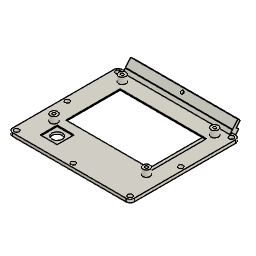
Display Mount Mini - LCD12864 Stock (Autodesk Fusion 360 design; units mm, degrees)
Autodesk Fusion 360 part; units mm, degrees
sketch "Sketch1" plane through (0, 0, 0) normal (0, 0, 1) x (1, 0, 0)
  line L0 (-57.9, 52.128) -> (57.9, 52.128)
  line L1 (57.9, 52.128) -> (57.9, -52.128)
  line L2 (57.9, -52.128) -> (-57.9, -52.128)
  line L3 (-57.9, -52.128) -> (-57.9, 52.128)
  circle A0 centre (-54, 48.228) radius 3.9
  circle A1 centre (-54, 0) radius 2.25
  circle A2 centre (-54, -48.228) radius 3.9
  circle A3 centre (0, -48.228) radius 2.25
  circle A4 centre (54, -48.228) radius 3.9
  circle A5 centre (54, 0) radius 2.25
  circle A6 centre (54, 48.228) radius 3.9
  circle A7 centre (-54, 48.228) radius 2.25
  circle A8 centre (-54, -48.228) radius 2.25
  circle A9 centre (54, -48.228) radius 2.25
  circle A10 centre (54, 48.228) radius 2.25
  point P0 (0, 52.128)
  point P1 (-57.9, 0)
  dimension "d1" = 115.8
  dimension "d2" = 104.256
  dimension "d3" = 7.8
  dimension "d4" = 7.8
  dimension "d5" = 7.8
  dimension "d6" = 7.8
  dimension "d7" = 4.5
  dimension "d8" = 4.5
  dimension "d9" = 4.5
  dimension "d10" = 4.5
  dimension "d11" = 4.5
  dimension "d12" = 4.5
  dimension "d13" = 4.5
  dimension "d14" = 48.128
  dimension "d15" = 96.256
  dimension "d16" = 53.9
  dimension "d17" = 107.8
  constraint horizontal L0
  constraint vertical L1
  constraint horizontal L2
  constraint vertical L3
  constraint midpoint L0 P0
  constraint midpoint L3 P1
  constraint vertical origin P0
  constraint horizontal origin P1
  constraint concentric A0 A7
  constraint concentric A2 A8
  constraint concentric A4 A9
  constraint concentric A6 A10
  constraint tangent L0 A0
  constraint tangent L3 A0
  constraint tangent L1 A4
  constraint tangent L2 A4
  constraint horizontal A0.centre A6.centre
  constraint vertical A5.centre A6.centre
  constraint vertical A5.centre A4.centre
  constraint horizontal A3.centre A2.centre
  constraint horizontal A3.centre A4.centre
  constraint vertical A1.centre A0.centre
  constraint vertical A1.centre A2.centre
  constraint horizontal origin A1.centre
  constraint horizontal origin A5.centre
  constraint vertical origin A3.centre
  measures "d1" distance of L1.end L2.end
  measures "d2" distance of L0.end L1.end
  measures "d3" diameter of A0
  measures "d4" diameter of A2
  measures "d5" diameter of A4
  measures "d6" diameter of A6
  measures "d7" diameter of A1
  measures "d8" diameter of A5
  measures "d9" diameter of A3
  measures "d10" diameter of A7
  measures "d11" diameter of A8
  measures "d12" diameter of A9
  measures "d13" diameter of A10
extrude "Extrude1" add sketch "Sketch1" along normal blind 3 contours L0 L1 L2 L3 A0 A2 A4 A6 | A0 | A6 | A2 | A4
sketch "Sketch2" plane through (0, 0, 0) normal (1, 0, 0) x (0, 1, 0)
  line L0 (-2.25, 3) -> (2.25, 3)
  line L1 (-50.478, 3) -> (-45.978, 3)
  line L2 (-2.25, 3) -> (2.25, 3)
  line L3 (45.978, 3) -> (50.478, 3)
  line L4 (-50.478, 3) -> (-45.978, 3)
  line L5 (45.978, 3) -> (50.478, 3)
  line L6 (-50.478, 3) -> (-45.978, 3)
  line L7 (-48.228, 3) -> (-52.128, 3)
  line L8 (-48.228, 3) -> (48.228, 3)
  line L9 (52.128, 3) -> (48.228, 3)
  line L10 (52.128, 3) -> (48.228, 3)
  line L11 (48.228, 3) -> (-48.228, 3)
  line L12 (-48.228, 3) -> (-52.128, 3)
  line L13 (52.128, 0) -> (52.128, 3)
  line L14 (52.128, 3) -> (52.128, 0)
  line L15 (-2.25, 0) -> (2.25, 0)
  line L16 (-50.478, 0) -> (-45.978, 0)
  line L17 (-2.25, 0) -> (2.25, 0)
  line L18 (45.978, 0) -> (50.478, 0)
  line L19 (-50.478, 0) -> (-45.978, 0)
  line L20 (45.978, 0) -> (50.478, 0)
  line L21 (-50.478, 0) -> (-45.978, 0)
  line L22 (-48.228, 0) -> (-52.128, 0)
  line L23 (-48.228, 0) -> (-52.128, 0)
  line L24 (-48.228, 0) -> (48.228, 0)
  line L25 (52.128, 0) -> (48.228, 0)
  line L26 (52.128, 0) -> (48.228, 0)
  line L27 (48.228, 0) -> (-48.228, 0)
  line L28 (52.128, 3) -> (52.128, 6)
  line L29 (52.128, 6) -> (55.128, 6)
  line L30 (55.128, 6) -> (58.0826, 3.5208)
  line L31 (58.0826, 3.5208) -> (56.1543, 1.2226)
  line L32 (56.1543, 1.2226) -> (62.2826, -3.9197)
  line L33 (62.2826, -3.9197) -> (61.2567, -5.1423)
  line L34 (61.2567, -5.1423) -> (55.1284, 0)
  line L35 (56.1543, 1.2226) -> (55.1284, 0)
  line L36 (55.1284, 0) -> (52.128, 0)
  dimension "d20" = 3
  dimension "d21" = 3
  dimension "d22" = 140
  dimension "d24" = 3.857
  dimension "d26" = 3
  dimension "d27" = 8
  dimension "d28" = 1.596
  constraint coincident L9.start L10.start
  constraint perpendicular L10 L28
  constraint perpendicular L28 L29
  constraint perpendicular L30 L31
  constraint perpendicular L31 L32
  constraint perpendicular L32 L33
  constraint perpendicular L33 L34
  constraint collinear L31 L35
  constraint coincident L13.start L14.end
  measures "d20" distance of L9.start L28.end
  measures "d21" distance of L28.end L29.end
  measures "d22" angle of L29 L30
  measures "d24" distance of L29.end L30.end
  measures "d26" distance of L30.end L31.end
  measures "d27" distance of L31.end L32.end
  measures "d28" distance of L32.end L33.end
extrude "Extrude2" add sketch "Sketch2" along normal mid plane 102 contours L13 L14 L28 L29 L30 L31 L35 L36
sketch "Sketch1 (2)" plane through (0, 25.732, 30.6662) normal (0, 0.642788, 0.766044) x (-1, 0, 0)
  line L0 (51, -38.3738) -> (-51, -38.3738)
  line L1 (-51, -38.3738) -> (-51, -42.2308)
  line L2 (-51, -42.2308) -> (51, -42.2308)
  line L3 (51, -42.2308) -> (51, -38.3738)
  line L4 (51, -39.2308) -> (-51, -39.2308)
  line L5 (-51, -39.2308) -> (-51, -36.2308)
  line L6 (-51, -36.2308) -> (51, -36.2308)
  line L7 (51, -36.2308) -> (51, -39.2308)
  dimension "d67" = 3
  dimension "d68" = 3
  constraint horizontal L4
  constraint vertical L5
  constraint horizontal L6
  constraint vertical L7
  constraint collinear L1 L5
  constraint collinear L3 L7
  measures "d67" distance of L2 L4
  measures "d68" distance of L4 L6
extrude "Extrude4" add sketch "Sketch1 (2)" against normal blind 7 contours L0 L1 L3 L4 L5 L7 | L0 L5 L6 L7
sketch "Sketch2 (2)" plane through (0, 25.732, 30.6662) normal (0, 0.642788, 0.766044) x (-1, 0, 0)
  line L0 (-51, -36.2308) -> (-51, -42.2308)
  line L1 (-51, -42.2308) -> (51, -42.2308)
  line L2 (51, -42.2308) -> (51, -36.2308)
  line L3 (51, -36.2308) -> (-51, -36.2308)
  line L4 (51, -39.2308) -> (-51, -39.2308)
  line L5 (-51, -39.2308) -> (-51, -36.2308)
  line L6 (-51, -36.2308) -> (51, -36.2308)
  line L7 (51, -36.2308) -> (51, -39.2308)
  dimension "d71" = 3
  constraint horizontal L4
  constraint vertical L5
  constraint horizontal L6
  constraint vertical L7
  constraint coincident L0.start L3.end
  constraint coincident L2 L4.start
  measures "d71" distance of L1 L4
extrude "Extrude5" add sketch "Sketch2 (2)" along normal blind 6 contours L0 L2 L3 L4 L5 L6 L7
sketch "Sketch3" plane through (0, 30.0525, -25.2171) normal (0, 0.766044, -0.642788) x (-1, 0, 0)
  line L0 (-51, 40.0319) -> (51, 40.0319)
  line L1 (51, 40.0319) -> (51, 46.0319)
  line L2 (51, 46.0319) -> (-51, 46.0319)
  line L3 (-51, 46.0319) -> (-51, 40.0319)
  circle A0 centre (0, 43.0319) radius 1.425
  dimension "d74" = 2.85
  dimension "d75" = 3
  constraint vertical origin A0.centre
  measures "d74" diameter of A0
  measures "d75" distance of L2 A0.centre
extrude "Extrude6" cut sketch "Sketch3" against normal blind 4 contours A0
sketch "Sketch5" plane through (0, 0, 3) normal (0, 0, 1) x (-1, 0, 0)
  line L0 (-51, -52.128) -> (-51, -49.8132)
  line L1 (-51, -49.8132) -> (51, -49.8132)
  line L2 (51, -49.8132) -> (51, -52.128)
  line L3 (51, -52.128) -> (54, -52.128)
  arc A0 (54, -52.128) -> (57.9, -48.228) centre (54, -48.228) ccw
  line L4 (57.9, -48.228) -> (57.9, 48.228)
  arc A1 (57.9, 48.228) -> (54, 52.128) centre (54, 48.228) ccw
  line L5 (54, 52.128) -> (-54, 52.128)
  arc A2 (-54, 52.128) -> (-57.9, 48.228) centre (-54, 48.228) ccw
  line L6 (-57.9, 48.228) -> (-57.9, -48.228)
  arc A3 (-57.9, -48.228) -> (-54, -52.128) centre (-54, -48.228) ccw
  line L7 (-54, -52.128) -> (-51, -52.128)
  circle A4 centre (-54, 48.228) radius 2.25
  circle A5 centre (-54, -48.228) radius 2.25
  circle A6 centre (54, 48.228) radius 2.25
  circle A7 centre (54, -48.228) radius 2.25
  circle A8 centre (54, 0) radius 2.25
  circle A9 centre (0, 48.228) radius 2.25
  circle A10 centre (-54, 0) radius 2.25
  line L8 (49.9, -44.128) -> (-49.9, -44.128)
  line L9 (-49.9, -44.128) -> (-49.9, 44.128)
  line L10 (-49.9, 44.128) -> (49.9, 44.128)
  line L11 (49.9, 44.128) -> (49.9, -44.128)
  dimension "d84" = 8
  dimension "d85" = 8
  dimension "d86" = 8
  dimension "d87" = 8
  constraint horizontal L8
  constraint vertical L9
  constraint horizontal L10
  constraint vertical L11
  measures "d84" distance of L4 L11
  measures "d85" distance of L6 L9
  measures "d86" distance of L5 L10
  measures "d87" distance of L2.end L8
extrude "Extrude7" add sketch "Sketch5" along normal blind 6 contours L8 L9 L10 L11
fillet "Fillet1" radius 3 4 edges at (-49.9, -44.128, 6) (-49.9, 44.128, 6) (49.9, -44.128, 6) (49.9, 44.128, 6)
sketch "Sketch4" plane through (0, 0, 9) normal (0, 0, 1) x (-1, 0, 0)
  line L0 (-51, -52.128) -> (-51, -49.8132)
  line L1 (-51, -49.8132) -> (51, -49.8132)
  line L2 (51, -49.8132) -> (51, -52.128)
  line L3 (51, -52.128) -> (54, -52.128)
  arc A0 (54, -52.128) -> (57.9, -48.228) centre (54, -48.228) ccw
  line L4 (57.9, -48.228) -> (57.9, 48.228)
  arc A1 (57.9, 48.228) -> (54, 52.128) centre (54, 48.228) ccw
  line L5 (54, 52.128) -> (-54, 52.128)
  arc A2 (-54, 52.128) -> (-57.9, 48.228) centre (-54, 48.228) ccw
  line L6 (-57.9, 48.228) -> (-57.9, -48.228)
  arc A3 (-57.9, -48.228) -> (-54, -52.128) centre (-54, -48.228) ccw
  line L7 (-54, -52.128) -> (-51, -52.128)
  circle A4 centre (-54, 48.228) radius 2.25
  circle A5 centre (-54, -48.228) radius 2.25
  circle A6 centre (54, 48.228) radius 2.25
  circle A7 centre (54, -48.228) radius 2.25
  circle A8 centre (54, 0) radius 2.25
  circle A9 centre (0, 48.228) radius 2.25
  circle A10 centre (-54, 0) radius 2.25
  line L8 (0, -78.513) -> (0, 73.0042) construction
  line L9 (78.1431, -3) -> (75.8671, -3)
  line L10 (75.8671, -3) -> (-80.0089, -3) construction
  line L11 (47.5, -50.3125) -> (-47.5, -50.3125)
  line L12 (-47.5, -50.3125) -> (-47.5, 44.3125)
  line L13 (-47.5, 44.3125) -> (47.5, 44.3125)
  line L14 (47.5, 44.3125) -> (47.5, -50.3125)
  line L15 (39, -35.25) -> (-39.2, -35.25)
  line L16 (-39.2, -35.25) -> (-39.2, 16.25)
  line L17 (-39.2, 16.25) -> (39, 16.25)
  line L18 (39, 16.25) -> (39, -35.25)
  line L19 (49.9, 41.128) -> (49.9, -41.128)
  arc A11 (46.9, -44.128) -> (49.9, -41.128) centre (46.9, -41.128) ccw
  line L20 (46.9, -44.128) -> (-46.9, -44.128)
  arc A12 (-49.9, -41.128) -> (-46.9, -44.128) centre (-46.9, -41.128) ccw
  line L21 (-49.9, -41.128) -> (-49.9, 41.128)
  arc A13 (-46.9, 44.128) -> (-49.9, 41.128) centre (-46.9, 41.128) ccw
  line L22 (-46.9, 44.128) -> (46.9, 44.128)
  arc A14 (49.9, 41.128) -> (46.9, 44.128) centre (46.9, 41.128) ccw
  arc A15 (-49.9, -41.128) -> (-46.9, -44.128) centre (-46.9, -41.128) ccw
  line L23 (-46.9, -44.128) -> (46.9, -44.128)
  arc A16 (46.9, -44.128) -> (49.9, -41.128) centre (46.9, -41.128) ccw
  line L24 (49.9, -41.128) -> (49.9, 41.128)
  arc A17 (49.9, 41.128) -> (46.9, 44.128) centre (46.9, 41.128) ccw
  line L25 (46.9, 44.128) -> (-46.9, 44.128)
  arc A18 (-46.9, 44.128) -> (-49.9, 41.128) centre (-46.9, 41.128) ccw
  line L26 (-49.9, 41.128) -> (-49.9, -41.128)
  circle A19 centre (44, -42.3125) radius 1.425
  circle A20 centre (44, -42.3125) radius 2.5 construction
  circle A21 centre (44, -42.3125) radius 3.5
  circle A22 centre (-44, -42.3125) radius 1.425
  circle A23 centre (-44, -42.3125) radius 2.5 construction
  circle A24 centre (-44, -42.3125) radius 3.5
  line L27 (40.5, -50.3125) -> (40.5, -42.3125)
  line L28 (44, -38.8125) -> (47.5, -38.8125)
  line L29 (-40.5, -42.3125) -> (-40.5, -45.727)
  line L30 (-40.5, -45.727) -> (-40.5, -50.3125)
  line L31 (-44, -38.8125) -> (-44.8157, -38.8125)
  line L32 (-44.8157, -38.8125) -> (-47.5, -38.8125)
  circle A25 centre (44, 22.6875) radius 1.425
  circle A26 centre (44, 22.6875) radius 2.5 construction
  circle A27 centre (44, 22.6875) radius 3.5
  circle A28 centre (-44, 22.6875) radius 1.425
  circle A29 centre (-44, 22.6875) radius 2.5 construction
  circle A30 centre (-44, 22.6875) radius 3.5
  line L33 (41.5251, 25.1624) -> (47.5, 31.1372)
  line L34 (41.5251, 25.1624) -> (50.2544, 25.1624) construction
  line L35 (41.5251, 20.2126) -> (47.5, 14.2378)
  line L36 (41.5251, 20.2126) -> (51.4571, 20.2126) construction
  line L37 (-41.5251, 25.1624) -> (-47.5, 31.1372)
  line L38 (-41.5251, 20.2126) -> (-47.5, 14.2378)
  circle A31 centre (31, 32.678) radius 5
  line L39 (39, 24.678) -> (23, 24.678)
  line L40 (23, 24.678) -> (23, 40.678)
  line L41 (23, 40.678) -> (39, 40.678)
  line L42 (39, 40.678) -> (39, 24.678)
  line L43 (39, 24.678) -> (23, 40.678) construction
  point P0 (0, -50.3125)
  dimension "d78" = 95
  dimension "d79" = 94.625
  dimension "d80" = 39
  dimension "d81" = 78.2
  dimension "d82" = 19.25
  dimension "d83" = 51.5
  dimension "d92" = 47.3125
  dimension "d93" = 47.3125
  dimension "d94" = 14.0625
  dimension "d95" = 3
  dimension "d96" = 2.85
  dimension "d97" = 5
  dimension "d98" = 7
  dimension "d99" = 8
  dimension "d100" = 2.85
  dimension "d101" = 5
  dimension "d103" = 7
  dimension "d104" = 2.85
  dimension "d105" = 5
  dimension "d106" = 7
  dimension "d107" = 2.85
  dimension "d108" = 5
  dimension "d109" = 7
  dimension "d110" = 65
  dimension "d111" = 45
  dimension "d113" = 45
  dimension "d115" = 45
  dimension "d116" = 45
  dimension "d117" = 10
  dimension "d118" = 16
  dimension "d119" = 16
  dimension "d120" = 16.5
  dimension "d121" = 11.45
  constraint perpendicular L5 L8
  constraint horizontal L9
  constraint perpendicular L6 L10
  constraint coincident origin L8
  constraint horizontal L11
  constraint vertical L12
  constraint horizontal L13
  constraint vertical L14
  constraint midpoint L11 P0
  constraint vertical origin P0
  constraint horizontal L15
  constraint vertical L16
  constraint horizontal L17
  constraint vertical L18
  constraint concentric A19 A20
  constraint concentric A20 A21
  constraint tangent L14 A21
  constraint concentric A22 A23
  constraint concentric A23 A24
  constraint tangent L12 A24
  constraint horizontal A19.centre A22.centre
  constraint coincident L11 L27.start
  constraint coincident A21 L27.end
  constraint perpendicular L11 L27
  constraint tangent A21 L27
  constraint coincident A21 L28.start
  constraint coincident L14 L28.end
  constraint tangent A21 L28
  constraint perpendicular L14 L28
  constraint coincident A24 L29.start
  constraint tangent A24 L29
  constraint perpendicular L1 L29
  constraint coincident L11 L30.end
  constraint perpendicular L11 L30
  constraint coincident A24 L31.start
  constraint tangent A24 L31
  constraint perpendicular L12 L31
  constraint coincident L12 L32.end
  constraint perpendicular L12 L32
  constraint concentric A25 A26
  constraint concentric A26 A27
  constraint concentric A28 A29
  constraint concentric A29 A30
  constraint tangent L12 A30
  constraint tangent L14 A27
  constraint horizontal A25.centre A28.centre
  constraint horizontal L34
  constraint coincident A27 L33.start
  constraint tangent A27 L33
  constraint horizontal L36
  constraint coincident A27 L35.start
  constraint tangent A27 L35
  constraint coincident L14 L35.end
  constraint coincident L14 L33.end
  constraint coincident A30 L37.start
  constraint coincident L12 L37.end
  constraint coincident A30 L38.start
  constraint coincident L12 L38.end
  constraint tangent A30 L38
  constraint tangent A30 L37
  constraint horizontal L39
  constraint vertical L40
  constraint horizontal L41
  constraint vertical L42
  constraint coincident A31.centre L43
  constraint midpoint A31.centre L43
  measures "d78" distance of L11.start L11.end
  measures "d79" distance of L11.end L12.end
  measures "d80" distance of L8 L18
  measures "d81" distance of L16 L18
  measures "d82" distance of L10 L17
  measures "d83" distance of L15 L17
  measures "d92" distance of L10 L13
  measures "d93" distance of L10 L11
  measures "d95" distance of origin L10
  measures "d96" diameter of A19
  measures "d97" diameter of A20
  measures "d98" diameter of A21
  measures "d99" distance of L11 A19.centre
  measures "d100" diameter of A22
  measures "d101" diameter of A23
  measures "d103" diameter of A24
  measures "d104" diameter of A25
  measures "d105" diameter of A26
  measures "d106" diameter of A27
  measures "d107" diameter of A28
  measures "d108" diameter of A29
  measures "d109" diameter of A30
  measures "d110" distance of A19.centre A25.centre
  measures "d111" angle of L33 L34
  measures "d113" angle of L35 L36
  measures "d115" angle of L12 L38
  measures "d116" angle of L12 L37
  measures "d117" diameter of A31
  measures "d118" distance of L39.start L39.end
  measures "d119" distance of L39.start L41.end
  measures "d120" distance of L14 A31.centre
  measures "d121" distance of L22 A31.centre
extrude "Extrude9" cut sketch "Sketch4" against normal blind 8.5 contours A19 | A22
extrude "Extrude8" add sketch "Sketch4" against normal blind 8 contours L20 A12 A15 L23 A24 | A11 L20 L23 A16 A21 picked at (-43.0708, -44.2671) picked at (43.0708, -44.2671)
extrude "Extrude10" cut sketch "Sketch4" against normal blind 10 contours L15 L16 L17 L18
extrude "Extrude11" cut sketch "Sketch4" against normal up to surface (6 mm away) contours A25 | A28
extrude "Extrude13" cut sketch "Sketch4" against normal blind 7 contours L39 L40 L41 L42
extrude "Extrude14" cut sketch "Sketch4" against normal through all contours A31
extrude "Extrude15" cut sketch "Sketch4" against normal blind 6 contours L12 A12 L21 A13 A15 A18 L26 | L12 A12 A15 A24 | L12 A24 L31 L32 | L20 L23 A21 L27 | L12 L14 L20 A13 L22 A14 L23 A17 L25 A18 A21 A24 L27 L28 L29 L31 L32 A27 A30 L33 L35 L37 L38 | L20 L23 A24 L29 | L14 A11 A16 A21 | L14 L19 A11 A14 A16 L24 A17 | L12 A30 L38 | L14 A21 L28 | L12 A30 L37 | L14 A27 L35 | L14 A27 L33
chamfer "Chamfer1" distance 2 angle 45 4 edges at (39.2, 9.5, 0) (0.1, 35.25, 0) (-39, 9.5, 0) (0.1, -16.25, 0)
sketch "Sketch6" plane through (0, 0, 3) normal (0, 0, 1) x (-1, 0, 0)
  line L0 (-51, -52.128) -> (-51, -49.8132)
  line L1 (-51, -49.8132) -> (51, -49.8132)
  line L2 (51, -49.8132) -> (51, -52.128)
  line L3 (51, -52.128) -> (54, -52.128)
  arc A0 (54, -52.128) -> (57.9, -48.228) centre (54, -48.228) ccw
  line L4 (57.9, -48.228) -> (57.9, 48.228)
  arc A1 (57.9, 48.228) -> (54, 52.128) centre (54, 48.228) ccw
  line L5 (54, 52.128) -> (-54, 52.128)
  arc A2 (-54, 52.128) -> (-57.9, 48.228) centre (-54, 48.228) ccw
  line L6 (-57.9, 48.228) -> (-57.9, -48.228)
  arc A3 (-57.9, -48.228) -> (-54, -52.128) centre (-54, -48.228) ccw
  circle A4 centre (-54, 48.228) radius 2.25
  circle A5 centre (-54, -48.228) radius 2.25
  circle A6 centre (54, 48.228) radius 2.25
  circle A7 centre (54, -48.228) radius 2.25
  circle A8 centre (54, 0) radius 2.25
  circle A9 centre (0, 48.228) radius 2.25
  circle A10 centre (-54, 0) radius 2.25
  line L7 (-39.2, -35.25) -> (-43.2, -35.25)
  line L8 (-43.2, -35.25) -> (-43.2, 16.25)
  line L9 (-43.2, 16.25) -> (-39.2, 16.25)
  line L10 (-39.2, 16.25) -> (-39.2, -35.25)
  circle A11 centre (-44, -42.3125) radius 3.5
  circle A12 centre (-44, 22.6875) radius 3.5
  line L11 (-39.2, 16.25) -> (39, 16.25)
  line L12 (39, 16.25) -> (39, -35.25)
  line L13 (39, -35.25) -> (-39.2, -35.25)
  line L14 (-39.2, -35.25) -> (-39.2, 16.25)
  circle A13 centre (44, 22.6875) radius 3.5
  line L15 (23, 40.678) -> (39, 40.678)
  line L16 (39, 40.678) -> (39, 24.678)
  line L17 (39, 24.678) -> (23, 24.678)
  line L18 (23, 24.678) -> (23, 40.678)
  circle A14 centre (44, -42.3125) radius 3.5
  line L19 (-54, -52.128) -> (-51, -52.128)
  dimension "d139" = 4
  constraint horizontal L7
  constraint vertical L8
  constraint horizontal L9
  constraint vertical L10
  measures "d139" distance of L8 L10
extrude "Extrude16" cut sketch "Sketch6" against normal blind 1 contours L7 L8 L9 L10 L14
equation "d4 = d3"
equation "d5 = d3"
equation "d6 = d3"
equation "d8 = d7"
equation "d9 = d7"
equation "d10 = d7"
equation "d11 = d7"
equation "d12 = d7"
equation "d13 = d7"
equation "d119 = d118"
